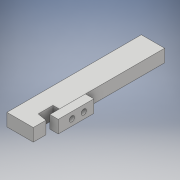
# Autodesk Inventor part: RimKey
Saved by Autodesk Inventor 2018 (Build 220112000, 112)
## iProperties
Created: 2018-01-20
Part Number: RimKey
Material: Generic
Document SubType Name: Modeling
Designer: eroldan
Density: 1 g/cm^3
Appearance: Default
Author: eroldan
Autodesk Inventor part; units mm, degrees
ref_plane "YZ Plane" through (0, 0, 0) normal (1, 0, 0) x (0, 1, 0)
ref_plane "XZ Plane" through (0, 0, 0) normal (0, 1, 0) x (-1, 0, 0)
ref_plane "XY Plane" through (0, 0, 0) normal (0, 0, 1) x (1, 0, 0)
sketch "Sketch1" plane through (0, 0, 0) normal (0, 0, 1) x (1, 0, 0)
  line L0 (0, 0) -> (0, 127.5628)
  line L1 (0, 127.5628) -> (22.1367, 127.5628)
  line L2 (22.1367, 27.5628) -> (16.1367, 27.5628)
  line L3 (16.1367, 27.5628) -> (16.1367, 13.5628)
  line L4 (25, 12) -> (25, 0)
  line L5 (25, 0) -> (0, 0)
  line L6 (22.1367, 127.5628) -> (22.1367, 27.5628)
  line L7 (16.1367, 13.5628) -> (25, 12)
  dimension "d1" = 14
  dimension "d2" = 6
  dimension "d3" = 12
  dimension "d4" = 100
  dimension "d5" = 9
  dimension "d6" = 25
  dimension "d9" = 100
  constraints: 16 end point, 3 perpendicular, 2 vertical, 1 horizontal
  measures "d1" distance of L2.end L3.end
  measures "d2" distance of L2.start L2.end
  measures "d3" distance of L4.start L4.end
  measures "d4" angle of L3 L7
  measures "d5" distance of L3.end L4.start
  measures "d6" distance of L4.end L0.start
  measures "d9" distance of L1.end L2.start
extrude "Extrusion1" add sketch "Sketch1" along normal blind 12
sketch "Sketch2" plane through (22.1367, 27.5628, 0) normal (1, 0, 0) x (0, 0, -1)
  line L0 (0, 0) -> (-12, 0) construction
  line L1 (-12, 24.8201) -> (0, 24.8201)
  line L2 (0, 24.8201) -> (0, -9)
  line L3 (0, -9) -> (-12, -9)
  line L4 (-12, -9) -> (-12, 24.8201)
  line L5 (-6, 0) -> (-6, 34.7527) construction
  circle A0 centre (-6, 15.2194) radius 2.5
  circle A1 centre (-6, 3.9579) radius 2.5
  point P0 (0, -27.5628)
  dimension "d11" = 9
  dimension "d12" = 5
  dimension "d13" = 5
  constraints: 10 end point, 2 centre point, 2 parallel, 2 point on line, 1 horizontal, 1 midpoint, 1 perpendicular, 1 vertical
  measures "d11" distance between parallel lines of L0 L3
  measures "d12" diameter of A0
  measures "d13" diameter of A1
extrude "Extrusion2" add sketch "Sketch2" along normal blind 8 separate body
sketch "Sketch3" plane through (0, 0, 0) normal (-1, 0, 0) x (0, 0, 1)
  circle A0 centre (6, 42.7823) radius 2.5 projected
  circle A1 centre (6, 31.5207) radius 2.5 projected
  point P0 (0, 0)
hole "Hole1" at (0, 31.5207, 6) at (0, 42.7823, 6) direction (1, 0, 0) diameter 5 end through all bodies 1
body "Solid1"
body "Solid2"
